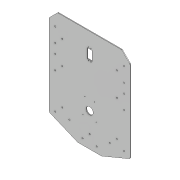
# Autodesk Inventor part: top
Saved by Autodesk Inventor 2020 (Build 240168000, 168)
## iProperties
Created: 2020-09-06
Part Number: top
Material: 알루미늄 6061-AHC
Document SubType Name: Sheet Metal
Designer: 이호석
Mass: 1109.06 g
Surface Area: 2799.86 cm^2
Volume: 410.763 cm^3
Density: 2.7 g/cm^3
Sheet Metal Rule: 기본값_mm
Appearance: 알루미늄 - 짙음
Flat Pattern Width: 34 cm
Flat Pattern Length: 43 cm
Flat Pattern Area: 1462 cm^2
Sheet Metal Width: 340.000 mm
Sheet Metal Length: 430.000 mm
Sheet Metal Area: 146200.000 mm^2
Author: 이호석
Autodesk Inventor part; units mm, degrees
ref_plane "YZ Plane" through (0, 0, 0) normal (1, 0, 0) x (0, 1, 0)
ref_plane "XZ Plane" through (0, 0, 0) normal (0, 1, 0) x (-1, 0, 0)
ref_plane "XY Plane" through (0, 0, 0) normal (0, 0, 1) x (1, 0, 0)
sketch "스케치1" plane through (0, 0, 0) normal (0, 0, 1) x (1, 0, 0)
  line L0 (50, -215) -> (-50, -215)
  line L1 (-170, -165) -> (-170, 179.6447)
  line L2 (-134.6447, 215) -> (134.6447, 215)
  line L3 (170, 179.6447) -> (170, -165)
  line L4 (-170, -165) -> (-50, -215)
  line L5 (170, -165) -> (50, -215)
  line L6 (-134.6447, 215) -> (-170, 179.6447)
  line L7 (134.6447, 215) -> (170, 179.6447)
extrude "판1" add sketch "스케치1" along normal blind 3
sketch "스케치3" plane through (0, 0, 3) normal (0, 0, 1) x (1, 0, 0)
  line L0 (50, -215) -> (-50, -215) projected
  line L1 (0, -215) -> (0, -75)
  line L2 (0, -75) -> (0, -102.87)
  line L3 (0, -75) -> (0, -33)
  line L4 (-20, -33) -> (20, -33)
  line L5 (-28, -102.87) -> (28, -102.87)
  circle A0 centre (-20, -33) radius 1.35
  circle A1 centre (20, -33) radius 1.35
  circle A2 centre (-28, -102.87) radius 1.35
  circle A3 centre (28, -102.87) radius 1.35
  circle A4 centre (0, -75) radius 15
  line L6 (0, -102.87) -> (-28, -102.87)
  line L7 (0, -33) -> (-20, -33)
  dimension "d32" = 140
  dimension "d34" = 27.87
  dimension "d35" = 42
  dimension "d37" = 40
  dimension "d39" = 56
  dimension "d40" = 2.7
  dimension "d41" = 2.7
  dimension "d42" = 2.7
  dimension "d43" = 2.7
  dimension "d44" = 30
  constraints: 14 end point, 6 coincident, 5 centre point, 2 collinear, 2 vertical, 1 midpoint, 1 point on line
  measures "d32" distance of L1.start L1.end
  measures "d34" distance of L2.start L2.end
  measures "d35" distance of L2.start L3.end
  measures "d37" distance of L4.start L4.end
  measures "d39" distance of L5.start L5.end
  measures "d40" diameter of A0
  measures "d41" diameter of A1
  measures "d42" diameter of A2
  measures "d43" diameter of A3
  measures "d44" diameter of A4
extrude "돌출2" cut sketch "스케치3" against normal through all
fillet "모서리 라운드1" radius 6 8 edges at (-134.6447, 215, 1.5) (-170, 179.6447, 1.5) (134.6447, 215, 1.5) (170, 179.6447, 1.5) (170, -165, 1.5) (50, -215, 1.5) (-50, -215, 1.5) (-170, -165, 1.5)
sketch "스케치4" plane through (0, 0, 3) normal (0, 0, 1) x (1, 0, 0)
  line L0 (48.8, -215) -> (-48.8, -215)
  line L1 (0, -215) -> (0, -205)
  line L2 (0, -205) -> (-15, -205)
  line L3 (-15, -205) -> (15, -205)
  line L4 (15, -205) -> (15, -175)
  line L5 (15, -175) -> (-15, -175)
  line L6 (-15, -175) -> (-15, -205)
  line L7 (130, -125) -> (130, 15)
  line L8 (-130, -125) -> (-130, 15)
  line L9 (-130, 15) -> (-160, 15)
  line L10 (-160, 15) -> (-160, 45)
  line L11 (-160, 45) -> (-130, 45)
  line L12 (-130, 45) -> (-130, 15)
  line L13 (130, 15) -> (160, 15)
  line L14 (160, 15) -> (160, 45)
  line L15 (160, 45) -> (130, 45)
  line L16 (130, 45) -> (130, 15)
  line L17 (130, 45) -> (130, 115)
  line L18 (-130, 45) -> (-130, 115)
  line L19 (-130, 115) -> (-160, 115)
  line L20 (-160, 115) -> (-160, 145)
  line L21 (-160, 145) -> (-130, 145)
  line L22 (-130, 145) -> (-130, 115)
  line L23 (130, 115) -> (160, 115)
  line L24 (160, 115) -> (160, 145)
  line L25 (160, 145) -> (130, 145)
  line L26 (130, 145) -> (130, 115)
  line L27 (165, -125) -> (170, -125)
  line L28 (170, -125) -> (170, -25)
  line L29 (170, -25) -> (165, -25)
  line L30 (165, -25) -> (165, -125)
  line L31 (-165, -125) -> (-170, -125)
  line L32 (-170, -125) -> (-170, -25)
  line L33 (-170, -25) -> (-165, -25)
  line L34 (-165, -25) -> (-165, -125)
  line L35 (-170, -125) -> (-170, -75)
  line L36 (-170, -161) -> (-170, 177.1594)
  line L37 (-170, -75) -> (170, -75)
  line L38 (0, -215) -> (0, -165)
  line L39 (0, -165) -> (-130, -165)
  line L40 (0, -165) -> (130, -165)
  line L41 (130, -165) -> (100, -165)
  line L42 (100, -165) -> (100, -135)
  line L43 (100, -135) -> (130, -135)
  line L44 (130, -135) -> (130, -165)
  line L45 (-130, -165) -> (-100, -165)
  line L46 (-100, -165) -> (-100, -135)
  line L47 (-100, -135) -> (-130, -135)
  line L48 (-130, -135) -> (-130, -165)
  line L49 (130, -135) -> (130, -125)
  line L50 (130, -125) -> (165, -125)
  line L51 (-130, -135) -> (-130, -125)
  line L52 (-130, -125) -> (-165, -125)
  line L53 (-100, -165) -> (-100, -162.5)
  line L54 (-100, -135) -> (-102.5, -135)
  line L55 (-130, -135) -> (-130, -137.5)
  line L56 (100, -165) -> (100, -162.5)
  line L57 (100, -135) -> (102.5, -135)
  line L58 (130, -135) -> (130, -137.5)
  line L59 (-15, -205) -> (-15, -202.5)
  line L60 (-15, -175) -> (-12.5, -175)
  line L61 (15, -175) -> (15, -177.5)
  line L62 (-130, -137.5) -> (-160, -137.5)
  line L63 (-160, -137.5) -> (-160, -162.5)
  line L64 (-160, -162.5) -> (-130, -162.5)
  line L65 (-130, -162.5) -> (-130, -137.5)
  line L66 (-102.5, -135) -> (-127.5, -135)
  line L67 (-127.5, -135) -> (-127.5, -105)
  line L68 (-127.5, -105) -> (-102.5, -105)
  line L69 (-102.5, -105) -> (-102.5, -135)
  line L70 (-100, -162.5) -> (-70, -162.5)
  line L71 (-70, -162.5) -> (-70, -137.5)
  line L72 (-70, -137.5) -> (-100, -137.5)
  line L73 (-100, -137.5) -> (-100, -162.5)
  line L74 (-12.5, -175) -> (12.5, -175)
  line L75 (12.5, -175) -> (12.5, -145)
  line L76 (12.5, -145) -> (-12.5, -145)
  line L77 (-12.5, -145) -> (-12.5, -175)
  line L78 (-15, -202.5) -> (-45, -202.5)
  line L79 (-45, -202.5) -> (-45, -177.5)
  line L80 (-45, -177.5) -> (-15, -177.5)
  line L81 (-15, -177.5) -> (-15, -202.5)
  line L82 (15, -177.5) -> (45, -177.5)
  line L83 (45, -177.5) -> (45, -202.5)
  line L84 (45, -202.5) -> (15, -202.5)
  line L85 (15, -202.5) -> (15, -177.5)
  line L86 (100, -162.5) -> (70, -162.5)
  line L87 (70, -162.5) -> (70, -137.5)
  line L88 (70, -137.5) -> (100, -137.5)
  line L89 (100, -137.5) -> (100, -162.5)
  line L90 (102.5, -135) -> (127.5, -135)
  line L91 (127.5, -135) -> (127.5, -105)
  line L92 (127.5, -105) -> (102.5, -105)
  line L93 (102.5, -105) -> (102.5, -135)
  line L94 (130, -137.5) -> (160, -137.5)
  line L95 (160, -137.5) -> (160, -162.5)
  line L96 (160, -162.5) -> (130, -162.5)
  line L97 (130, -162.5) -> (130, -137.5)
  line L98 (0, -175) -> (0, -160)
  line L99 (-15, -205) -> (-15, -190)
  line L100 (-15, -190) -> (-30, -190)
  line L101 (15, -190) -> (30, -190)
  line L102 (-100, -165) -> (-100, -150)
  line L103 (-100, -150) -> (-85, -150)
  line L104 (-130, -150) -> (-145, -150)
  line L105 (-115, -135) -> (-115, -120)
  line L106 (100, -165) -> (100, -150)
  line L107 (100, -150) -> (85, -150)
  line L108 (130, -165) -> (130, -150)
  line L109 (130, -150) -> (145, -150)
  line L110 (127.5, -135) -> (115, -135)
  line L111 (115, -135) -> (115, -120)
  circle A0 centre (-85, -150) radius 2.6
  circle A1 centre (-145, -150) radius 2.6
  circle A2 centre (-115, -120) radius 2.6
  circle A3 centre (-30, -190) radius 2.6
  circle A4 centre (30, -190) radius 2.6
  circle A5 centre (0, -160) radius 2.6
  circle A6 centre (85, -150) radius 2.6
  circle A7 centre (115, -120) radius 2.6
  circle A8 centre (145, -150) radius 2.6
  line L112 (-130, 15) -> (-145, 15)
  line L113 (-145, 15) -> (-145, 0)
  line L114 (130, 15) -> (145, 15)
  line L115 (145, 15) -> (145, 0)
  line L116 (-145, 45) -> (-145, 60)
  line L117 (-145, 115) -> (-145, 100)
  line L118 (-145, 145) -> (-145, 160)
  line L119 (145, 45) -> (145, 60)
  line L120 (145, 115) -> (145, 100)
  line L121 (145, 145) -> (145, 160)
  line L122 (130, 145) -> (130, 130)
  line L123 (130, 130) -> (115, 130)
  line L124 (-130, 130) -> (-115, 130)
  line L125 (-130, 30) -> (-115, 30)
  line L126 (130, 30) -> (115, 30)
  circle A9 centre (145, 0) radius 2.6
  circle A10 centre (115, 30) radius 2.6
  circle A11 centre (145, 60) radius 2.6
  circle A12 centre (145, 100) radius 2.6
  circle A13 centre (115, 130) radius 2.6
  circle A14 centre (145, 160) radius 2.6
  circle A15 centre (-145, 100) radius 2.6
  circle A16 centre (-115, 130) radius 2.6
  circle A17 centre (-145, 160) radius 2.6
  circle A18 centre (-145, 60) radius 2.6
  circle A19 centre (-115, 30) radius 2.6
  circle A20 centre (-145, 0) radius 2.6
  point P0 (0, 0)
  point P1 (0, 0)
  dimension "d48" = 2.5
  dimension "d49" = 2.5
  dimension "d50" = 2.5
  dimension "d51" = 2.5
  dimension "d52" = 2.5
  dimension "d53" = 2.5
  dimension "d54" = 2.5
  dimension "d55" = 2.5
  dimension "d56" = 2.5
  dimension "d57" = 30
  dimension "d58" = 25
  dimension "d59" = 25
  dimension "d60" = 30
  dimension "d61" = 30
  dimension "d62" = 25
  dimension "d63" = 25
  dimension "d64" = 30
  dimension "d65" = 30
  dimension "d66" = 25
  dimension "d67" = 30
  dimension "d68" = 25
  dimension "d69" = 30
  dimension "d70" = 25
  dimension "d71" = 25
  dimension "d72" = 30
  dimension "d73" = 30
  dimension "d74" = 25
  dimension "d75" = 15
  dimension "d76" = 15
  dimension "d77" = 15
  dimension "d78" = 15
  dimension "d79" = 15
  dimension "d80" = 15
  dimension "d81" = 15
  dimension "d82" = 5.2
  dimension "d83" = 5.2
  dimension "d84" = 5.2
  dimension "d85" = 5.2
  dimension "d86" = 5.2
  dimension "d87" = 5.2
  dimension "d88" = 5.2
  dimension "d89" = 5.2
  dimension "d90" = 15
  dimension "d91" = 15
  dimension "d92" = 15
  dimension "d93" = 15
  dimension "d94" = 15
  dimension "d95" = 15
  dimension "d96" = 15
  dimension "d97" = 15
  dimension "d98" = 15
  dimension "d99" = 15
  dimension "d100" = 15
  dimension "d101" = 15
  dimension "d102" = 15
  dimension "d103" = 5.2
  dimension "d104" = 5.2
  dimension "d105" = 5.2
  dimension "d106" = 5.2
  dimension "d107" = 5.2
  constraints: 254 end point, 36 parallel, 30 perpendicular, 24 horizontal, 23 midpoint, 21 centre point, 21 coincident, 15 vertical, 11 point on line
  measures "d48" distance of L45.end L53.end
  measures "d49" distance of L46.end L54.end
  measures "d50" distance of L47.end L55.end
  measures "d51" distance of L41.end L56.end
  measures "d52" distance of L42.end L57.end
  measures "d53" distance of L43.end L58.end
  measures "d54" distance of L2.end L59.end
  measures "d55" distance of L5.end L60.end
  measures "d56" distance of L4.end L61.end
  measures "d57" distance of L64.end L63.end
  measures "d58" distance of L63.end L62.end
  measures "d59" distance of L67.end L68.end
  measures "d60" distance of L66.end L67.end
  measures "d61" distance of L72.end L71.end
  measures "d62" distance of L71.end L70.end
  measures "d63" distance of L76.end L75.end
  measures "d64" distance of L75.end L74.end
  measures "d65" distance of L79.end L80.end
  measures "d66" distance of L78.end L79.end
  measures "d67" distance of L83.end L84.end
  measures "d68" distance of L82.end L83.end
  measures "d69" distance of L87.end L88.end
  measures "d70" distance of L86.end L87.end
  measures "d71" distance of L92.end L91.end
  measures "d72" distance of L91.end L90.end
  measures "d73" distance of L95.end L96.end
  measures "d74" distance of L94.end L95.end
  measures "d75" distance of L98.start L98.end
  measures "d76" distance of L2.end L99.end
  measures "d77" distance of L99.end L100.end
  measures "d78" distance of L101.start L101.end
  measures "d79" distance of L105.start L105.end
  measures "d80" distance of L41.end L106.end
  measures "d81" distance of L106.end L107.end
  measures "d82" diameter of A0
  measures "d83" diameter of A2
  measures "d84" diameter of A3
  measures "d85" diameter of A4
  measures "d86" diameter of A5
  measures "d87" diameter of A6
  measures "d88" diameter of A7
  measures "d89" diameter of A8
  measures "d90" distance of L8.end L112.end
  measures "d91" distance of L112.end L113.end
  measures "d92" distance of L7.end L114.end
  measures "d93" distance of L116.start L116.end
  measures "d94" distance of L117.start L117.end
  measures "d95" distance of L118.start L118.end
  measures "d96" distance of L119.start L119.end
  measures "d97" distance of L120.start L120.end
  measures "d98" distance of L121.start L121.end
  measures "d99" distance of L25.end L122.end
  measures "d100" distance of L122.end L123.end
  measures "d101" distance of L124.start L124.end
  measures "d102" distance of L126.start L126.end
  measures "d103" diameter of A9
  measures "d104" diameter of A10
  measures "d105" diameter of A11
  measures "d106" diameter of A12
  measures "d107" diameter of A14
extrude "돌출3" cut sketch "스케치4" against normal through all contours A0 | A1 | A2 | A3 | A4 | A5 | A6 | A7 | A8 | A9 | A10 | A11 | A12 | A13 | A14 | A15 | A16 | A17 | A18 | A19 | A20
sketch "스케치5" plane through (0, 0, 3) normal (0, 0, 1) x (1, 0, 0)
  circle A0 centre (-85, -150) radius 2.6 projected
  circle A1 centre (85, -150) radius 2.6 projected
  circle A2 centre (-145, 60) radius 2.6 projected
  circle A3 centre (-115, 30) radius 2.6 projected
  circle A4 centre (-145, 0) radius 2.6 projected
  circle A5 centre (145, 160) radius 2.6 projected
  circle A6 centre (145, 60) radius 2.6 projected
  circle A7 centre (115, 30) radius 2.6 projected
  circle A8 centre (115, -120) radius 2.6 projected
  circle A9 centre (-30, -190) radius 2.6 projected
  circle A10 centre (-115, -120) radius 2.6 projected
  circle A11 centre (30, -190) radius 2.6 projected
  circle A12 centre (-145, 100) radius 2.6 projected
  circle A13 centre (-115, 130) radius 2.6 projected
  circle A14 centre (145, 0) radius 2.6 projected
  circle A15 centre (-145, 160) radius 2.6 projected
  circle A16 centre (145, 100) radius 2.6 projected
  circle A17 centre (115, 130) radius 2.6 projected
  circle A18 centre (145, -150) radius 2.6 projected
  circle A19 centre (0, -160) radius 2.6 projected
  circle A20 centre (-145, -150) radius 2.6 projected
  arc A21 (-170, -161) -> (-166.3077, -166.5385) centre (-164, -161) ccw projected
  line L0 (-51.1077, -214.5385) -> (-166.3077, -166.5385) projected
  arc A22 (-51.1077, -214.5385) -> (-48.8, -215) centre (-48.8, -209) ccw projected
  line L1 (48.8, -215) -> (-48.8, -215) projected
  arc A23 (48.8, -215) -> (51.1077, -214.5385) centre (48.8, -209) ccw projected
  line L2 (166.3077, -166.5385) -> (51.1077, -214.5385) projected
  arc A24 (166.3077, -166.5385) -> (170, -161) centre (164, -161) ccw projected
  line L3 (170, 177.1594) -> (170, -161) projected
  arc A25 (170, 177.1594) -> (168.2426, 181.402) centre (164, 177.1594) ccw projected
  line L4 (136.402, 213.2426) -> (168.2426, 181.402) projected
  arc A26 (136.402, 213.2426) -> (132.1594, 215) centre (132.1594, 209) ccw projected
  line L5 (-132.1594, 215) -> (132.1594, 215) projected
  arc A27 (-132.1594, 215) -> (-136.402, 213.2426) centre (-132.1594, 209) ccw projected
  line L6 (-168.2426, 181.402) -> (-136.402, 213.2426) projected
  arc A28 (-168.2426, 181.402) -> (-170, 177.1594) centre (-164, 177.1594) ccw projected
  line L7 (-170, -161) -> (-170, 177.1594) projected
  circle A29 centre (-20, -33) radius 1.35 projected
  circle A30 centre (-28, -102.87) radius 1.35 projected
  circle A31 centre (20, -33) radius 1.35 projected
  circle A32 centre (28, -102.87) radius 1.35 projected
  circle A33 centre (0, -75) radius 15 projected
  line L8 (0, 0) -> (0, 130)
  line L9 (10.1, 150.1) -> (-10.1, 150.1)
  line L10 (-10.1, 150.1) -> (-10.1, 109.9)
  line L11 (-10.1, 109.9) -> (10.1, 109.9)
  line L12 (10.1, 109.9) -> (10.1, 150.1)
  line L13 (10.1, 150.1) -> (-10.1, 109.9) construction
  line L14 (-10.1, 150.1) -> (10.1, 109.9) construction
  line L15 (-10.1, 150.1) -> (-10.1, 154.75)
  line L16 (-10.1, 154.75) -> (-5.1, 154.75)
  line L17 (-5.1, 154.75) -> (4.9, 154.75)
  line L18 (-10.1, 109.9) -> (-10.1, 105.25)
  line L19 (-10.1, 105.25) -> (-5.1, 105.25)
  line L20 (-5.1, 105.25) -> (4.9, 105.25)
  circle A34 centre (4.9, 105.25) radius 1.6
  circle A35 centre (-5.1, 105.25) radius 1.6
  circle A36 centre (4.9, 154.75) radius 1.6
  circle A37 centre (-5.1, 154.75) radius 1.6
  dimension "d110" = 130
  dimension "d111" = 20.2
  dimension "d112" = 40.2
  dimension "d113" = 4.65
  dimension "d114" = 5
  dimension "d115" = 10
  dimension "d116" = 4.65
  dimension "d117" = 5
  dimension "d118" = 3.2
  constraints: 26 end point, 4 centre point, 4 coincident, 3 perpendicular, 3 vertical, 2 midpoint, 2 parallel, 2 point on line, 1 horizontal
  measures "d110" distance of L8.start L8.end
  measures "d111" distance of L11.end L10.end
  measures "d112" distance of L10.end L9.end
  measures "d113" distance of L9.end L15.end
  measures "d114" distance of L15.end L16.end
  measures "d115" distance of L16.end L17.end
  measures "d116" distance of L10.end L18.end
  measures "d117" distance of L18.end L19.end
  measures "d118" diameter of A34
extrude "돌출4" cut sketch "스케치5" against normal through all contours L11 L10 L9 L12 | A35 L19 L20 | L20 L19 A35 | A37 L17 L16 | L16 L17 A37 | A34 | A36
equation "\"TransitionRadius\" = BendRadius"
equation "\"BendRadius\" = 3"
